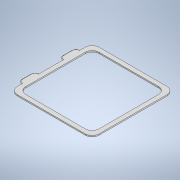
# Autodesk Inventor part: Plate
Saved by Autodesk Inventor 2020 (Build 240168000, 168)
## iProperties
Created: 2020-06-10
Part Number: Plate
Material: Generic
Document SubType Name: Modeling
Designer: maple
Density: 1 g/cm^3
Appearance: Default
Author: maple
Autodesk Inventor part; units mm, degrees
ref_plane "YZ Plane" through (0, 0, 0) normal (1, 0, 0) x (0, 1, 0)
ref_plane "XZ Plane" through (0, 0, 0) normal (0, 1, 0) x (-1, 0, 0)
ref_plane "XY Plane" through (0, 0, 0) normal (0, 0, 1) x (1, 0, 0)
sketch "Sketch1" plane through (0, 0, 0) normal (0, 1, 0) x (-1, 0, 0)
  line L0 (0, 0) -> (-95, 0)
  line L1 (-95, 0) -> (-95, -95)
  line L2 (-95, -95) -> (0, -95)
  line L3 (0, -95) -> (0, 0)
  line L4 (0, 0) -> (-5, 0)
  line L5 (-5, 0) -> (-5, -5)
  line L6 (-5, -5) -> (0, -5)
  line L7 (0, -5) -> (0, 0)
  line L8 (-95, -95) -> (-90, -95)
  line L9 (-90, -95) -> (-90, -90)
  line L10 (-90, -90) -> (-95, -90)
  line L11 (-95, -90) -> (-95, -95)
  line L12 (-90, -90) -> (-5, -90)
  line L13 (-5, -90) -> (-5, -5)
  line L14 (-5, -5) -> (-90, -5)
  line L15 (-90, -5) -> (-90, -90)
  line L16 (0, -47.5) -> (0, 0)
  line L17 (0, -47.5) -> (0, -95)
  line L18 (0, -23.75) -> (0, -18.75)
  line L19 (0, -18.75) -> (0, -28.75)
  line L20 (0, -71.25) -> (0, -76.25)
  line L21 (0, -76.25) -> (0, -66.25)
  line L22 (0, -18.75) -> (0, -28.75) construction
  line L23 (-5, -18.75) -> (-5, -28.75)
  line L24 (5, -28.75) -> (5, -18.75)
  arc A0 (5, -18.75) -> (-5, -18.75) centre (0, -18.75) ccw
  arc A1 (-5, -28.75) -> (5, -28.75) centre (0, -28.75) ccw
  line L25 (0, -66.25) -> (0, -76.25) construction
  line L26 (-5, -66.25) -> (-5, -76.25)
  line L27 (5, -76.25) -> (5, -66.25)
  arc A2 (5, -66.25) -> (-5, -66.25) centre (0, -66.25) ccw
  arc A3 (-5, -76.25) -> (5, -76.25) centre (0, -76.25) ccw
  point P0 (0, -61.25)
  point P1 (0, -81.25)
  point P2 (0, -13.75)
  point P3 (0, -33.75)
  dimension "d0" = 95
  dimension "d1" = 95
  dimension "d2" = 5
  dimension "d3" = 5
  dimension "d4" = 5
  dimension "d5" = 5
  dimension "d8" = 5
  dimension "d9" = 10
  dimension "d10" = 5
  dimension "d11" = 10
  dimension "d12" = 10
  dimension "d13" = 10
  constraints: 60 end point, 10 parallel, 8 point on circle, 8 tangent, 5 midpoint, 4 centre point, 4 collinear, 4 horizontal, 4 perpendicular, 4 point on line
  measures "d0" distance of L2.end L1.end
  measures "d1" distance of L1.end L0.end
  measures "d2" distance of L6.end L5.end
  measures "d3" distance of L5.end L4.end
  measures "d4" distance of L10.end L9.end
  measures "d5" distance of L9.end L8.end
  measures "d8" distance of L18.start L18.end
  measures "d9" distance of L18.end L19.end
  measures "d10" distance of L20.start L20.end
  measures "d11" distance of L20.end L21.end
  measures "d12" diameter of A1
  measures "d13" diameter of A3
extrude "Extrusion1" add sketch "Sketch1" along normal blind 1.5 contours L3 L6 L5 L0 | L5 L14 L15 L10 L1 L0 | L3 A0 L13 L6 | A0 L24 A1 L3 | L3 A1 L13 A0 | L10 L9 L2 L1 | L12 L13 A3 L3 L2 L9 | A1 L3 A2 L13 | A2 L3 A3 L13 | A2 L27 A3 L3
fillet "Fillet1" radius 8 8 edges at (5, 0.75, -5) (0, 0.75, 0) (0, 0.75, -95) (5, 0.75, -90) (95, 0.75, 0) (90, 0.75, -5) (95, 0.75, -95) (90, 0.75, -90)
fillet "Fillet2" radius 1 12 edges at (-3.5355, 0, -15.2145) (-3.5355, 0, -32.2855) (-5, 0, -23.75) (-3.5355, 1.5, -15.2145) (-3.5355, 1.5, -32.2855) (-5, 1.5, -23.75) (-3.5355, 0, -62.7145) (-3.5355, 0, -79.7855) (-5, 0, -71.25) (-3.5355, 1.5, -62.7145) (-3.5355, 1.5, -79.7855) (-5, 1.5, -71.25)
body "Solid1"
